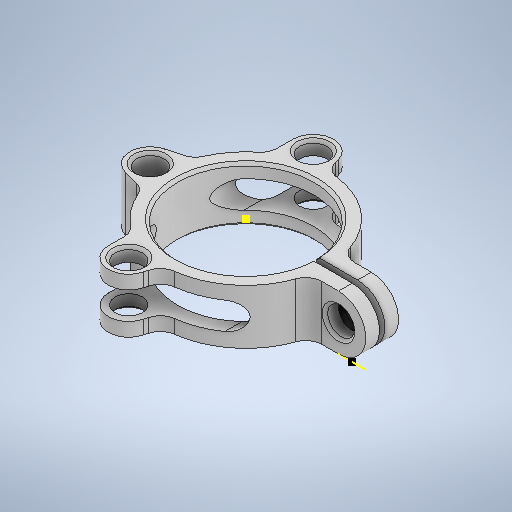
# Autodesk Inventor part: 19th_jianjeong_01
Saved by Autodesk Inventor 2025.1 (Build 291241000, 241)
## iProperties
Created: 2024-08-06
Part Number: 19th_jianjeong_01
Material: 일반
Document SubType Name: Modeling
Designer: naru4
Density: 1 g/cm^3
Appearance: 기본값
Author: naru4
Autodesk Inventor part; units mm, degrees
ref_plane "YZ Plane" through (0, 0, 0) normal (1, 0, 0) x (0, 1, 0)
ref_plane "XZ Plane" through (0, 0, 0) normal (0, 1, 0) x (-1, 0, 0)
ref_plane "XY Plane" through (0, 0, 0) normal (0, 0, 1) x (1, 0, 0)
sketch "스케치1" plane through (0, 0, 0) normal (0, 1, 0) x (-1, 0, 0)
  line L0 (0, 0) -> (35, 0) construction
  line L1 (0, 0) -> (35, 0) construction
  arc A0 (16.5587, 33.8074) -> (1.8142, 35.7485) centre (9.0587, 33.8074) ccw
  arc A1 (1.8142, -35.7485) -> (16.5587, -33.8074) centre (9.0587, -33.8074) ccw
  line L2 (0, 0) -> (35, 0)
  arc A2 (36.9411, -7.2444) -> (36.9411, 7.2444) centre (35, 0) ccw
  line L3 (0, 0) -> (-50, 0)
  line L4 (-50, 0) -> (-50, -6)
  line L5 (-50, -6) -> (-33.9411, -6)
  line L6 (-50, 0) -> (-50, 6)
  line L7 (-50, 6) -> (-33.9411, 6)
  line L8 (-50, 0) -> (-40, 0)
  circle A3 centre (9.0587, 33.8074) radius 5
  circle A4 centre (35, 0) radius 5
  circle A5 centre (9.0587, -33.8074) radius 5
  arc A6 (27.4484, 12.1073) -> (18.7989, 23.3795) centre (0, 0) ccw
  arc A7 (18.7989, -23.3795) -> (27.4484, -12.1073) centre (0, 0) ccw
  line L9 (16.5587, -33.8074) -> (16.5587, -28.0554)
  line L10 (36.9411, -7.2444) -> (31.3852, -8.7332)
  line L11 (36.9411, 7.2444) -> (31.3852, 8.7332)
  line L12 (16.5587, 33.8074) -> (16.5587, 28.0554)
  line L13 (1.8142, -35.7485) -> (1.3931, -34.1769)
  arc A8 (31.3852, -8.7332) -> (27.4484, -12.1073) centre (32.9381, -14.5287) ccw
  arc A9 (18.7989, -23.3795) -> (16.5587, -28.0554) centre (22.5587, -28.0554) ccw
  arc A10 (-3.6687, 29.7748) -> (-28.2843, 10) centre (0, 0) ccw
  arc A11 (-28.2843, -10) -> (-3.6687, -29.7748) centre (0, 0) ccw
  arc A12 (1.3931, -34.1769) -> (-3.6687, -29.7748) centre (-4.4025, -35.7298) ccw
  arc A13 (-28.2843, -10) -> (-33.9411, -6) centre (-33.9411, -12) ccw
  arc A14 (-33.9411, 6) -> (-28.2843, 10) centre (-33.9411, 12) ccw
  line L14 (1.8142, 35.7485) -> (1.3931, 34.1769)
  arc A15 (-3.6687, 29.7748) -> (1.3931, 34.1769) centre (-4.4025, 35.7298) ccw
  arc A16 (27.4484, 12.1073) -> (31.3852, 8.7332) centre (32.9381, 14.5287) ccw
  arc A17 (16.5587, 28.0554) -> (18.7989, 23.3795) centre (22.5587, 28.0554) ccw
  arc A18 (-24.98, -1) -> (-24.98, 1) centre (0, 0) ccw
  line L15 (-50, 0) -> (-50, -1)
  line L16 (-50, -1) -> (-50, 1)
  line L17 (-50, 1) -> (-24.98, 1)
  line L18 (-50, -1) -> (-24.98, -1)
  point P0 (-29.3939, 6)
  point P1 (16.5587, -25.0162)
  point P2 (28.4495, -9.5198)
  point P3 (0.2736, -29.9988)
  point P4 (28.4495, 9.5198)
  point P5 (-29.3939, -6)
  point P6 (-0.4651, -31.2024)
  point P7 (34.1631, 7.9888)
  dimension "d5" = 15
  dimension "d6" = 15
  dimension "d7" = 35
  dimension "d8" = 15
  dimension "d9" = 50
  dimension "d10" = 6
  dimension "d11" = 6
  dimension "d12" = 10
  dimension "d13" = 10
  dimension "d14" = 10
  dimension "d15" = 10
  dimension "d16" = 6
  dimension "d17" = 6
  dimension "d19" = 6
  dimension "d20" = 50
  dimension "d21" = 1
  dimension "d22" = 2
  constraints: 39 point on circle, 38 end point, 19 centre point, 19 tangent, 12 point on line, 6 coincident, 6 horizontal, 4 equal radius, 2 vertical, 1 midpoint, 10 other
  measures "d5" diameter of A0
  measures "d6" diameter of A1
  measures "d7" distance of L0.start L1.end
  measures "d8" diameter of A2
  measures "d9" distance of L0.start L3.end
  measures "d10" distance of L3.end L4.end
  measures "d11" distance of L3.end L6.end
  measures "d12" distance of L3.end L8.end
  measures "d13" diameter of A3
  measures "d14" diameter of A4
  measures "d15" diameter of A5
  measures "d16" radius of A8
  measures "d17" radius of A12
  measures "d19" radius of A16
  measures "d20" diameter of A18
  measures "d21" distance of L3.end L15.end
  measures "d22" distance of L15.end L16.end
extrude "돌출1" add sketch "스케치1" along normal blind 20 contours L12 A17 A6 A16 L11 A2 L10 A8 A7 A9 L9 A1 L13 A12 A11 A13 L5 L4 L18 A18 L17 L6 L7 A14 A10 A15 L14 A0
sketch "스케치3" plane through (0, 20, 0) normal (0, 1, 0) x (1, 0, 0)
  point P0 (0, 0)
sketch "스케치4" plane through (33.9411, 0, 6) normal (0, 0, 1) x (1, 0, 0)
  line L0 (-8.9611, 20) -> (16.0589, 20) projected
  line L1 (0, 0) -> (16.0589, 0) projected
  line L2 (16.0589, 0) -> (6.0589, 0)
  line L3 (16.0589, 20) -> (6.0589, 20)
  arc A0 (6.0589, 0) -> (6.0589, 20) centre (6.0589, 10) ccw
  line L4 (16.0589, 20) -> (16.0589, 0)
  point P0 (-33.9411, 0)
  point P1 (16.0589, 10)
  dimension "d26" = 10
  constraints: 6 end point, 2 point on circle, 2 point on line, 2 tangent, 1 centre point, 1 horizontal, 1 vertical
  measures "d26" distance of L1.end L2.end
extrude "돌출2" cut sketch "스케치4" against normal blind 20 contours L0 L4 A0
sketch "스케치5" plane through (33.9411, 0, 6) normal (0, 0, 1) x (1, 0, 0)
  arc A0 (16.0589, 10) -> (6.0589, 20) centre (6.0589, 10) ccw projected
  line L0 (16.0589, 0) -> (-8.9611, 0) projected
  arc A1 (6.0589, 0) -> (16.0589, 10) centre (6.0589, 10) ccw
  line L1 (16.0589, 10) -> (16.0589, 0)
  line L2 (6.0589, 0) -> (16.0589, 0)
  point P0 (-33.9411, 0)
  constraints: 4 end point, 2 point on circle, 1 centre point, 1 horizontal, 1 point on line, 1 tangent, 1 vertical
extrude "돌출3" cut sketch "스케치5" against normal blind 20
sketch "스케치6" plane through (33.9411, 0, 6) normal (0, 0, 1) x (1, 0, 0)
  arc A0 (6.0589, 0) -> (6.0589, 20) centre (6.0589, 10) ccw projected
  line L0 (6.0589, 20) -> (6.0589, 10)
  circle A1 centre (6.0589, 10) radius 5
  point P0 (-33.9411, 0)
  dimension "d31" = 10
  constraints: 2 end point, 1 centre point, 1 coincident, 1 vertical
  measures "d31" diameter of A1
extrude "돌출4" cut sketch "스케치6" against normal blind 20
chamfer "모따기1" distance 1 angle 45 10 edges at (35, 10, 6) (35, 10, -6) (-25, 20, 0) (-30, 20, 0) (-4.0587, 20, -33.8074) (-4.0587, 20, 33.8074) (-4.0587, 0, 33.8074) (-25, 0, 0) (-30, 0, 0) (-4.0587, 0, -33.8074)
sketch "스케치7" plane through (33.9411, 0, -6) normal (0, 0, -1) x (-1, 0, 0)
  circle A0 centre (-6.0589, 10) radius 6 projected
  circle A1 centre (-6.0589, 10) radius 5 projected
  line L0 (16.9411, 5) -> (51.9411, 5)
  line L1 (51.9411, 15) -> (16.9411, 15)
  line L2 (51.9411, 15) -> (86.9411, 15) construction
  arc A2 (51.9411, 5) -> (51.9411, 15) centre (51.9411, 10) ccw
  arc A3 (16.9411, 15) -> (16.9411, 5) centre (16.9411, 10) ccw
  point P0 (33.9411, 0)
  constraints: 6 end point, 4 horizontal, 4 point on circle, 4 tangent, 2 centre point, 1 collinear, 2 other
extrude "돌출5" cut sketch "스케치7" along normal mid plane 400 contours A3 L1 A2 L0
sketch "스케치9" plane through (0, 0, 0) normal (0, -1, 0) x (1, 0, 0)
  line L0 (40, 1) -> (40, 6) projected
  line L1 (50, 6) -> (40, 6) projected
  point P0 (0, 0)
  point P1 (45, 6)
  constraints: 1 midpoint
